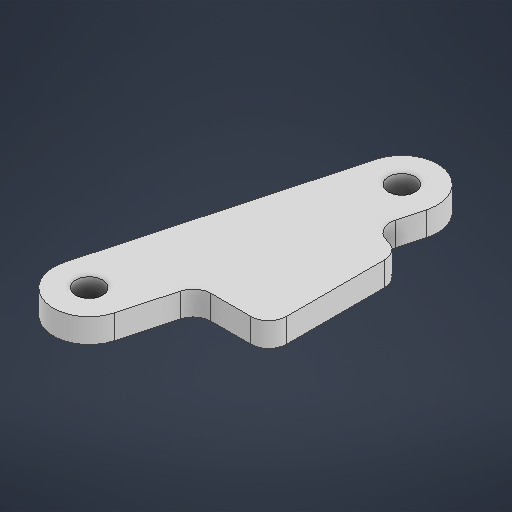
# Autodesk Inventor part: SujecionServo
Saved by Autodesk Inventor 2025.2 (Build 292293000, 293)
## iProperties
Created: 2025-10-07
Part Number: SujecionServo
Material: Generic
Document SubType Name: Modeling
Designer: Aarón Valerín
Density: 1 g/cm^3
Appearance: Default
Author: Aarón Valerín
Autodesk Inventor part; units mm, degrees
ref_plane "YZ Plane" through (0, 0, 0) normal (1, 0, 0) x (0, 1, 0)
ref_plane "XZ Plane" through (0, 0, 0) normal (0, 1, 0) x (-1, 0, 0)
ref_plane "XY Plane" through (0, 0, 0) normal (0, 0, 1) x (1, 0, 0)
sketch "Sketch1" plane through (0, 0, 0) normal (0, 1, 0) x (-1, 0, 0)
  line L0 (0, -3) -> (-10, -3)
  circle A0 centre (-21.6, 10.775) radius 1.5
  line L1 (0, 35) -> (-45, 35)
  line L2 (0, 0) -> (0, 35)
  circle A1 centre (-29.1, -16.775) radius 1.5
  arc A2 (-17.7405, 9.7243) -> (-25.4595, 11.8257) centre (-21.6, 10.775) ccw
  arc A3 (-32.9595, -15.7243) -> (-25.2405, -17.8257) centre (-29.1, -16.775) ccw
  line L3 (-17.7405, 9.7243) -> (-25.2405, -17.8257)
  line L4 (-27.4538, 4.5) -> (-35.4538, 4.5)
  line L5 (-35.4538, 4.5) -> (-35.4538, -10.5)
  line L6 (-35.4538, -10.5) -> (-31.5373, -10.5)
  line L7 (-25.4595, 11.8257) -> (-27.4538, 4.5)
  line L8 (-31.5373, -10.5) -> (-32.9595, -15.7243)
  point P0 (-35.4538, -3)
  dimension "d0" = 10
  dimension "d1" = 3
  dimension "d2" = 13.775
  dimension "d3" = 3
  dimension "d7" = 45
  dimension "d8" = 35
  dimension "d9" = 23.4
  dimension "d10" = 3
  dimension "d11" = 13.775
  dimension "d12" = 15.9
  dimension "d13" = 2.5
  dimension "d14" = 2.5
  dimension "d15" = 15
  dimension "d16" = 8
  constraints: 18 end point, 6 tangent, 4 centre point, 4 point on circle, 3 horizontal, 2 coincident, 2 perpendicular, 1 midpoint, 1 point on line, 1 vertical
  measures "d0" distance of L0.start L0.end
  measures "d1" distance from line of L0 L2.start
  measures "d2" distance from line of L0 A0.centre
  measures "d3" diameter of A0
  measures "d7" distance of L1.start L1.end
  measures "d8" distance from line of L2.start L1
  measures "d9" horizontal distance of A0.centre L1.end
  measures "d10" diameter of A1
  measures "d11" distance from line of L0 A1.centre
  measures "d12" horizontal distance of L1.end A1.centre
  measures "d13" radial gap between concentric circles of A2 A0
  measures "d14" radial gap between concentric circles of A3 A1
  measures "d15" distance of L4.end L5.end
  measures "d16" distance of L4.start L4.end
extrude "Extrusion1" add sketch "Sketch1" along normal blind 2.7
fillet "Fillet1" radius 2 4 edges at (35.4538, 1.35, 4.5) (27.4538, 1.35, 4.5) (35.4538, 1.35, -10.5) (31.5373, 1.35, -10.5)
body "Solid1"
